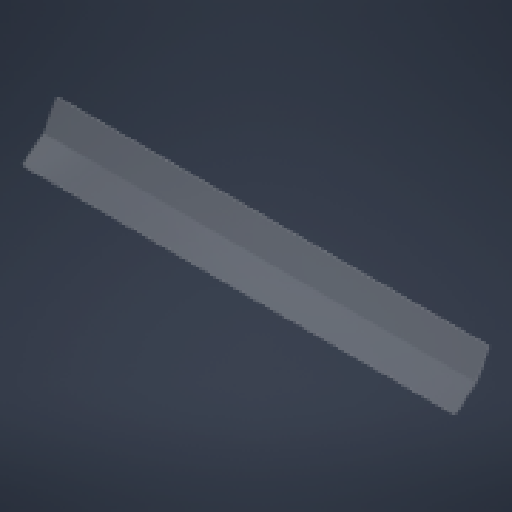
# Autodesk Inventor part: INTAKE,KICKER,PLATE
Saved by Autodesk Inventor 2026.2 (Build 302298010, 298A)
## iProperties
Created: 2026-04-02
Part Number: INTAKE,KICKER,PLATE
Material: Polycarbonate, Clear
Document SubType Name: Sheet Metal
Designer: Owen L
Density: 1.2 g/cm^3
Sheet Metal Rule: Default
Appearance: Polycarbonate - Clear
Author: Owen L
Autodesk Inventor part; units mm, degrees
note: some values were not read from the file. Chosen so that the rebuilt part matches the saved one: flange form of "Plate1".
ref_plane "YZ Plane" through (0, 0, 0) normal (1, 0, 0) x (0, 1, 0)
ref_plane "XZ Plane" through (0, 0, 0) normal (0, 1, 0) x (-1, 0, 0)
ref_plane "XY Plane" through (0, 0, 0) normal (0, 0, 1) x (1, 0, 0)
sketch "Sketch1" plane through (0, 0, 0) normal (1, 0, 0) x (0, 1, 0)
  line L0 (0, 0) -> (23.9771, -29.6093)
  line L1 (23.9771, -29.6093) -> (57.6174, -47.4961)
  line L2 (57.6174, -47.4961) -> (16.1556, -47.4961) construction
  dimension "d0" = 157
  dimension "d1" = 38.1
  dimension "d2" = 38.1
  dimension "d3" = 28
  measures "d0" angle of L1 L0
  measures "d1" distance of L0.start L0.end
  measures "d2" distance of L0.end L1.end
  measures "d3" angle of L1 L2
sketch "Sketch2" plane through (0, 0, 0) normal (0, 0.777146, 0.6293204) x (1, 0, 0)
  line L0 (5.5563, 3.175) -> (0, 3.175)
  line L1 (0, 3.175) -> (0, 13.175)
  line L2 (0, 13.175) -> (5.5563, 13.175)
  line L3 (5.5563, 13.175) -> (5.5563, 3.175)
  line L4 (583.2826, 0) -> (0, 0)
  line L5 (0, 0) -> (0, 37.454)
  line L6 (0, 30.6375) -> (5.5563, 30.6375)
  line L7 (5.5563, 30.6375) -> (5.5563, 20.6375)
  line L8 (5.5563, 20.6375) -> (0, 20.6375)
  line L9 (0, 20.6375) -> (0, 30.6375)
  line L10 (5.5562, 0) -> (5.5562, 37.454)
  line L11 (0, 37.454) -> (583.2826, 37.454)
  line L12 (0, 0) -> (583.2826, 0)
  line L13 (291.6413, 0) -> (291.6413, 37.454)
  line L14 (577.7263, 3.175) -> (583.2826, 3.175)
  line L15 (583.2826, 3.175) -> (583.2826, 13.175)
  line L16 (583.2826, 13.175) -> (577.7263, 13.175)
  line L17 (577.7263, 13.175) -> (577.7263, 3.175)
  line L18 (583.2826, 0) -> (583.2826, 37.454)
  line L19 (583.2826, 30.6375) -> (577.7263, 30.6375)
  line L20 (577.7263, 30.6375) -> (577.7263, 20.6375)
  line L21 (577.7263, 20.6375) -> (583.2826, 20.6375)
  line L22 (583.2826, 20.6375) -> (583.2826, 30.6375)
  line L23 (577.7263, 0) -> (577.7263, 37.454)
  line L24 (-3.175, 3.175) -> (-5.5563, 3.175)
  line L25 (-5.5563, 3.175) -> (-5.5563, 13.175)
  line L26 (-5.5563, 13.175) -> (-3.175, 13.175)
  line L27 (0, 13.175) -> (0, 3.175)
  line L28 (-3.175, 20.6375) -> (-5.5562, 20.6375)
  line L29 (-5.5562, 20.6375) -> (-5.5562, 30.6375)
  line L30 (-5.5562, 30.6375) -> (-3.175, 30.6375)
  line L31 (0, 30.6375) -> (0, 20.6375)
  line L32 (0, 16.35) -> (0, 17.4625)
  line L33 (0, 0) -> (0, 37.454)
  line L34 (0, 0) -> (0, 0)
  line L35 (0, 33.8125) -> (0, 37.454)
  arc A0 (0, 0) -> (-3.175, 3.175) centre (-3.175, 0) ccw
  arc A1 (-3.175, 13.175) -> (0, 16.35) centre (-3.175, 16.35) ccw
  arc A2 (0, 17.4625) -> (-3.175, 20.6375) centre (-3.175, 17.4625) ccw
  arc A3 (-3.175, 30.6375) -> (0, 33.8125) centre (-3.175, 33.8125) ccw
  line L36 (583.2826, 3.175) -> (583.2826, 13.175)
  line L37 (583.2826, 0) -> (583.2826, 37.454)
  line L38 (583.2826, 20.6375) -> (583.2826, 30.6375)
  line L39 (586.4576, 3.175) -> (588.8388, 3.175)
  line L40 (588.8388, 3.175) -> (588.8388, 13.175)
  line L41 (588.8388, 13.175) -> (586.4576, 13.175)
  line L42 (583.2826, 13.175) -> (583.2826, 3.175)
  line L43 (586.4576, 20.6375) -> (588.8388, 20.6375)
  line L44 (588.8388, 20.6375) -> (588.8388, 30.6375)
  line L45 (588.8388, 30.6375) -> (586.4576, 30.6375)
  line L46 (583.2826, 30.6375) -> (583.2826, 20.6375)
  line L47 (583.2826, 16.35) -> (583.2826, 17.4625)
  line L48 (583.2826, 0) -> (583.2826, 37.454)
  line L49 (583.2826, 0) -> (583.2826, 0)
  line L50 (583.2826, 33.8125) -> (583.2826, 37.454)
  arc A4 (586.4576, 3.175) -> (583.2826, 0) centre (586.4576, 0) ccw
  arc A5 (583.2826, 16.35) -> (586.4576, 13.175) centre (586.4576, 16.35) ccw
  arc A6 (586.4576, 20.6375) -> (583.2826, 17.4625) centre (586.4576, 17.4625) ccw
  arc A7 (583.2826, 33.8125) -> (586.4576, 30.6375) centre (586.4576, 33.8125) ccw
  point P0 (0, 17.4625)
  point P1 (0, 33.8125)
  point P2 (0, 0)
  point P3 (0, 3.175)
  point P4 (0, 13.175)
  point P5 (0, 16.35)
  point P6 (583.2826, 33.8125)
  point P7 (583.2826, 17.4625)
  point P8 (583.2826, 16.35)
  point P9 (583.2826, 0)
  dimension "d15" = 5.5563
  dimension "d16" = 10
  dimension "d17" = 3.175
  dimension "d18" = 7.4625
  dimension "d19" = 3.175
  dimension "d20" = 5.5563
  measures "d15" distance of L1.end L2.end
  measures "d16" distance of L1.end L0.end
  measures "d17" distance between parallel lines of L4 L0
  measures "d18" distance between parallel lines of L2 L8
  measures "d19" radius of A0
  measures "d20" distance between parallel lines of L1 L25
sketch "Sketch3" plane through (0, 57.6174, -47.4961) normal (0, 0.4694716, 0.8829476) x (1, 0, 0)
  line L0 (0, -30.6375) -> (0, -20.6375)
  line L1 (0, -37.454) -> (0, 0)
  line L2 (0, -13.175) -> (0, -3.175)
  line L3 (-3.175, -30.6375) -> (-5.5563, -30.6375)
  line L4 (-5.5563, -30.6375) -> (-5.5563, -20.6375)
  line L5 (-5.5563, -20.6375) -> (-3.175, -20.6375)
  line L6 (0, -20.6375) -> (0, -30.6375)
  line L7 (-3.175, -13.175) -> (-5.5563, -13.175)
  line L8 (-5.5563, -13.175) -> (-5.5563, -3.175)
  line L9 (-5.5563, -3.175) -> (-3.175, -3.175)
  line L10 (0, -3.175) -> (0, -13.175)
  line L11 (0, -17.4625) -> (0, -16.35)
  line L12 (0, -37.454) -> (0, 0)
  line L13 (0, -33.8125) -> (0, -37.454)
  line L14 (0, 0) -> (0, 0)
  arc A0 (0, -33.8125) -> (-3.175, -30.6375) centre (-3.175, -33.8125) ccw
  arc A1 (-3.175, -20.6375) -> (0, -17.4625) centre (-3.175, -17.4625) ccw
  arc A2 (0, -16.35) -> (-3.175, -13.175) centre (-3.175, -16.35) ccw
  arc A3 (-3.175, -3.175) -> (0, 0) centre (-3.175, 0) ccw
  line L15 (0, 0) -> (583.2826, 0)
  line L16 (291.6413, 0) -> (291.6413, -37.454)
  line L17 (0, -37.454) -> (583.2826, -37.454)
  line L18 (583.2826, -30.6375) -> (583.2826, -20.6375)
  line L19 (588.8388, -20.6375) -> (586.4576, -20.6375)
  line L20 (583.2826, -20.6375) -> (583.2826, -30.6375)
  line L21 (586.4576, -30.6375) -> (588.8388, -30.6375)
  line L22 (588.8388, -30.6375) -> (588.8388, -20.6375)
  line L23 (583.2826, -33.8125) -> (583.2826, -37.454)
  arc A4 (586.4576, -30.6375) -> (583.2826, -33.8125) centre (586.4576, -33.8125) ccw
  line L24 (583.2826, -37.454) -> (583.2826, 0)
  line L25 (583.2826, -13.175) -> (583.2826, -3.175)
  arc A5 (583.2826, -17.4625) -> (586.4576, -20.6375) centre (586.4576, -17.4625) ccw
  line L26 (586.4576, -13.175) -> (588.8388, -13.175)
  arc A6 (586.4576, -13.175) -> (583.2826, -16.35) centre (586.4576, -16.35) ccw
  line L27 (583.2826, -37.454) -> (583.2826, 0)
  line L28 (588.8388, -13.175) -> (588.8388, -3.175)
  line L29 (588.8388, -3.175) -> (586.4576, -3.175)
  line L30 (583.2826, -3.175) -> (583.2826, -13.175)
  arc A7 (583.2826, 0) -> (586.4576, -3.175) centre (586.4576, 0) ccw
  line L31 (583.2826, 0) -> (583.2826, 0)
  line L32 (583.2826, -17.4625) -> (583.2826, -16.35)
  line L33 (583.2826, 0) -> (583.2826, -33.8125)
  point P0 (0, -73.1712)
  point P1 (0, -33.8125)
  point P2 (0, -30.6375)
  point P3 (0, -20.6375)
  point P4 (0, -17.4625)
  point P5 (0, -16.35)
  point P6 (583.2826, -16.35)
  dimension "d26" = 10
  dimension "d27" = 3.175
  dimension "d28" = 5.5563
  dimension "d30" = 7.4625
  measures "d26" distance of L0.end L0.start
  measures "d27" radius of A0
  measures "d28" distance between parallel lines of L0 L4
  measures "d30" distance between parallel lines of L7 L5
contour flange "Contour Flange1" sketch "Sketch1" thickness 3.175 bend radius 3.175 width 583.2826 along (1, 0, 0) mid plane no both sides no wall seen from (0, 11.9886, -14.8046) lies toward (0, -0.777146, -0.6293204) curves L0 L1
bend "Bend1"
corner "Corner1"
sheet face with bend "Face1" sketch "Sketch2" thickness 3.175 toward (0, -0.777146, -0.6293204) bend radius 3.175 contours L5 A0 L24 L25 L26 A1 L1 | L5 A2 L28 L29 L30 A3 | L18 L15 A5 L41 L40 L39 A4 | A7 L45 L44 L43 A6 L18
bend "Bend2"
sheet face with bend "Face2" sketch "Sketch3" thickness 3.175 toward (0, -0.4694716, -0.8829476) bend radius 3.175 contours L1 A0 L3 L4 L5 A1 L0 | A2 L7 L8 L9 A3 L1 | A7 L29 L28 L26 A6 L24 | L24 L18 A5 L19 L22 L21 A4
bend "Bend3"
equation "\"d20\" = d15"
equation "\"d28\" = d29"
equation "\"d4\" = Thickness"
equation "\"d5\" = BendReliefWidth"
equation "\"d6\" = BendReliefDepth"
equation "\"d7\" = MinimumRemnant"
equation "\"d8\" = TransitionRadius"
equation "\"d10\" = BendRadius"
equation "\"d12\" = CornerReliefSize"
equation "\"d13\" = GapSize"
equation "\"d14\" = JacobiRadiusSize"
equation "\"d21\" = BendRadius"
equation "\"d22\" = BendReliefWidth"
equation "\"d24\" = MinimumRemnant"
equation "\"d23\" = BendReliefDepth"
equation "\"d25\" = TransitionRadius"
equation "\"d31\" = BendRadius"
equation "\"d32\" = BendReliefWidth"
equation "\"d34\" = MinimumRemnant"
equation "\"d33\" = BendReliefDepth"
equation "\"d35\" = TransitionRadius"
equation "\"BendRadius\" = Thickness"
equation "\"BendReliefWidth\" = Thickness"
equation "\"BendReliefDepth\" = 0.5 * Thickness"
equation "\"CornerReliefSize\" = 4 * Thickness"
equation "\"MinimumRemnant\" = 2 * Thickness"
equation "\"TransitionRadius\" = BendRadius"
equation "\"JacobiRadiusSize\" = BendRadius"
equation "\"GapSize\" = Thickness"
equation "\"d29\" = 5.55625"
equation "\"Thickness\" = 3.175"
body "Solid1"
